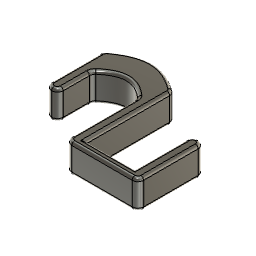
bag hook (Autodesk Fusion 360 design; units mm, degrees)
Autodesk Fusion 360 part; units mm, degrees
sketch "Sketch1" plane through (0, 0, 0) normal (0, 0, 1) x (1, 0, 0)
  line L0 (0, 0) -> (23, 0)
  line L1 (23, 0) -> (23, 20)
  line L2 (23, 20) -> (0, 20)
  line L3 (0, 20) -> (0, 0)
  line L4 (3, 0) -> (20, 0)
  line L5 (20, 0) -> (20, 17)
  line L6 (20, 17) -> (3, 17)
  line L7 (3, 17) -> (3, 0)
  line L8 (20, 0) -> (36, 0)
  line L9 (36, 0) -> (36, -13)
  line L10 (36, -13) -> (20, -13)
  line L11 (20, -13) -> (20, 0)
  line L12 (23, 0) -> (33, 0)
  line L13 (33, 0) -> (33, -10)
  line L14 (33, -10) -> (23, -10)
  line L15 (23, -10) -> (23, 0)
  line L16 (-10, 0) -> (-10, -13)
  line L17 (-10, -13) -> (-35, -13)
  line L18 (-35, -13) -> (-35, 0)
  line L19 (-14, 0) -> (-14, -10)
  line L20 (-14, -10) -> (-31, -10)
  line L21 (-31, -10) -> (-31, 0)
  line L22 (-35, 0) -> (-31, 0)
  line L23 (-14, 0) -> (-10, 0)
  line L24 (-31, 0) -> (-55, 0)
  line L25 (-55, 0) -> (-55, 20)
  line L26 (-55, 20) -> (-31, 20)
  line L27 (-31, 20) -> (-31, 0)
  line L28 (-35, 0) -> (-51, 0)
  line L29 (-51, 0) -> (-51, 16)
  line L30 (-51, 16) -> (-35, 16)
  line L31 (-35, 16) -> (-35, 0)
  spline S0 degree 5 poles (-31, 20) (-31.48, 20.3792) (-32.44, 21.1046) (-33.88, 22.0933) (-35.8, 23.2095) (-38.2, 24.2453) (-40.6, 24.8894) (-43, 25.11) (-45.4, 24.8894) (-47.8, 24.2453) (-50.2, 23.2095) (-52.12, 22.0933) (-53.56, 21.1046) (-54.52, 20.3792) (-55, 20) knots 0 0 0 0 0 0 0.1 0.2 0.3 0.4 0.5 0.6 0.7 0.8 0.9 1 1 1 1 1 1
  spline S1 degree 5 poles (-35, 12) (-35.32, 12.3034) (-35.96, 12.8837) (-36.92, 13.6746) (-38.2, 14.5676) (-39.8, 15.3962) (-41.4, 15.9116) (-43, 16.088) (-44.6, 15.9116) (-46.2, 15.3962) (-47.8, 14.5676) (-49.08, 13.6746) (-50.04, 12.8837) (-50.68, 12.3034) (-51, 12) knots 0 0 0 0 0 0 0.1 0.2 0.3 0.4 0.5 0.6 0.7 0.8 0.9 1 1 1 1 1 1
  line L32 (-10, 0) -> (-14, 0)
  line L33 (-14, 0) -> (-14, 10)
  line L34 (-14, 10) -> (-10, 10)
  line L35 (-10, 10) -> (-10, 0)
  point P0 (-43, 25)
  point P1 (-43, 16)
  dimension "d1" = 23
  dimension "d2" = 20
  dimension "d3" = 17
  dimension "d4" = 17
  dimension "d5" = 16
  dimension "d6" = 13
  dimension "d7" = 10
  dimension "d8" = 10
  dimension "d11" = 25
  dimension "d12" = 13
  dimension "d13" = 17
  dimension "d14" = 10
  dimension "d15" = 24
  dimension "d16" = 20
  dimension "d29" = 4
  dimension "d30" = 10
  constraint horizontal L0
  constraint vertical L1
  constraint horizontal L2
  constraint vertical L3
  constraint coincident L0.start L3.end
  constraint horizontal L4
  constraint vertical L5
  constraint horizontal L6
  constraint vertical L7
  constraint coincident L0 L4.start
  constraint horizontal L8
  constraint vertical L9
  constraint horizontal L10
  constraint vertical L11
  constraint horizontal L12
  constraint vertical L13
  constraint horizontal L14
  constraint vertical L15
  constraint horizontal L22
  constraint vertical L16
  constraint horizontal L17
  constraint vertical L18
  constraint vertical L19
  constraint horizontal L20
  constraint vertical L21
  constraint collinear L22 L23
  constraint horizontal L24
  constraint vertical L25
  constraint horizontal L26
  constraint vertical L27
  constraint horizontal L28
  constraint vertical L29
  constraint horizontal L30
  constraint vertical L31
  constraint coincident L31 S1.start
  constraint midpoint L30 P1
  constraint coincident L29 S1.end
  constraint horizontal L32
  constraint vertical L33
  constraint horizontal L34
  constraint vertical L35
  measures "d1" distance of L0.start L0.end
  measures "d2" distance of L0.start L2.end
  measures "d3" distance of L4.start L4.end
  measures "d4" distance of L4.start L6.end
  measures "d5" distance of L4.end L8.end
  measures "d6" distance of L4.end L10.end
  measures "d7" distance of L0.end L12.end
  measures "d8" distance of L0.end L14.end
  measures "d11" distance of L18.end L16.start
  measures "d12" distance of L18.end L17.end
  measures "d13" distance of L21.end L19.start
  measures "d14" distance of L21.end L20.end
  measures "d15" distance of L21.end L24.end
  measures "d16" distance of L21.end L26.end
  measures "d29" distance of L16.start L19.start
  measures "d30" distance of L16.start L34.end
extrude "Extrude3" add sketch "Sketch1" along normal blind 10 contours L16 L17 L18 L19 L20 L21 L22 L23 L24 L32 | L23 L32 L33 L34 L35 | L22 L24 L25 L26 L27 L29 L30 L31 | L30 L31 S1 | L26 S0 | L29 L30 S1
fillet "Fillet6" radius 2 10 edges at (-14, 10, 5) (-10, 10, 5) (-10, -13, 5) (-35, -13, 5) (-35, 12, 5) (-31, 20, 5) (-55, 20, 5) (-55, 0, 5) (-51, 0, 5) (-51, 12, 5)
fillet "Fillet7" radius 1 2 faces at (-32.3333, 6.7107, 10) (-32.3333, 6.7107, 0)
